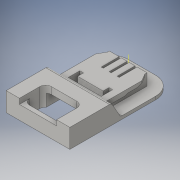
# Autodesk Inventor part: gehaeuse
Saved by Autodesk Inventor 2016 (Build 200138000, 138)
## iProperties
Created: 2016-06-09
Part Number: gehaeuse
Material: Generic
Document SubType Name: Modeling
Designer: Chris
Density: 1 g/cm^3
Appearance: Default
Author: Chris
Autodesk Inventor part; units mm, degrees
ref_plane "YZ Plane" through (0, 0, 0) normal (1, 0, 0) x (0, 1, 0)
ref_plane "XZ Plane" through (0, 0, 0) normal (0, 1, 0) x (-1, 0, 0)
sketch "Sketch1" plane through (0, 0, 0) normal (0, 0, 1) x (1, 0, 0)
  line L0 (-17.75, 0) -> (17.75, 0)
  line L1 (17.75, 0) -> (17.75, -85)
  line L2 (17.75, -85) -> (-17.75, -85)
  line L3 (-17.75, -85) -> (-17.75, 0)
  point P0 (0, 0)
  point P1 (0, 0)
  dimension "d0" = 35.5
  dimension "d1" = 85
  constraints: 8 end point, 2 parallel, 1 coincident, 1 horizontal, 1 midpoint, 1 perpendicular
  measures "d0" distance of L1.end L2.end
  measures "d1" distance of L0.end L1.end
extrude "Extrusion1" add sketch "Sketch1" along normal blind 11
sketch "Sketch2" plane through (0, 0, 0) normal (1, 0, 0) x (0, 1, 0)
  line L0 (-85, 0) -> (0, 0) projected
  line L1 (-85, 0) -> (-85, 11) projected
  line L2 (0, 11) -> (-85, 11) projected
  line L3 (0, 0) -> (0, 11) projected
  line L4 (-85, 82.7102) -> (-37.2472, 0)
  line L5 (0, 0) -> (0, 11) projected
  line L6 (0, 9) -> (-9, 9)
  line L7 (-9, 9) -> (-13.1212, 7.5)
  line L8 (-13.1212, 7.5) -> (-22, 7.5)
  line L9 (-22, 7.5) -> (-24.7475, 6.5)
  line L10 (-24.7475, 6.5) -> (-41, 6.5)
  line L11 (-45.9075, 15) -> (-85, 15)
  line L12 (-85, 15) -> (-85, 11)
  point P0 (-43.5981, 11)
  dimension "d6" = 60
  dimension "d7" = 20
  dimension "d8" = 2
  dimension "d9" = 3.5
  dimension "d10" = 4.5
  dimension "d11" = 6.5
  dimension "d12" = 9
  dimension "d13" = 13.1212
  dimension "d14" = 24.7475
  dimension "d15" = 22
  dimension "d16" = 41
  dimension "d25" = 15
  dimension "d26" = 4
  constraints: 16 end point, 8 point on line, 3 parallel, 3 perpendicular
  measures "d6" angle of L0 L4
  measures "d7" angle of L6 L7
  measures "d8" distance between parallel lines of L2 L6
  measures "d9" distance between parallel lines of L2 L8
  measures "d10" distance between parallel lines of L2 L10
  measures "d11" distance between parallel lines of L0 L10
  measures "d12" distance from line of L3 L6.end
  measures "d13" distance from line of L3 L7.end
  measures "d14" distance from line of L3 L9.end
  measures "d15" distance from line of L3 L8.end
  measures "d16" distance from line of L3 L10.end
  measures "d25" distance between parallel lines of L0 L11
  measures "d26" distance between parallel lines of L11 L2
extrude "Extrusion2" add sketch "Sketch2" along normal mid plane 60 contours L1 L2 L4 L0 | L12 L11 L4 L2
extrude "Extrusion4" add sketch "Sketch2" along normal mid plane 43.6 contours L4 L2 L3 L6 L7 L8 L9 L10
sketch "Sketch3" plane through (0, 0, 0) normal (0, 0, 1) x (1, 0, 0)
  line L0 (-13, 13) -> (13, 13)
  line L1 (-17.75, 0) -> (17.75, 0) projected
  line L2 (-30, -37.2472) -> (-30, -85) projected
  line L3 (30, -85) -> (30, -37.2472) projected
  line L4 (30, -85) -> (-30, -85) projected
  arc A0 (-13, 13) -> (-30, -4) centre (-13, -4) ccw
  arc A1 (30, -4) -> (13, 13) centre (13, -4) ccw
  line L5 (-30, -37.2472) -> (-30, -4)
  line L6 (30, -37.2472) -> (30, -4)
  point P0 (0, 0)
  dimension "d28" = 13
  dimension "d29" = 17
  constraints: 6 end point, 4 point on circle, 4 tangent, 2 centre point, 2 vertical, 1 equal radius, 1 horizontal
  measures "d28" distance between parallel lines of L0 L1
  measures "d29" radius of A0
extrude "Extrusion5" add sketch "Sketch3" against normal blind 3
fillet "Fillet1" radius 3 1 edges at (0, -45.9075, 15)
fillet "Fillet2" radius 2 2 edges at (23.875, -37.2472, 0) (-23.875, -37.2472, 0)
sketch "Sketch4" plane through (0, 0, 11) normal (0, 0, 1) x (1, 0, 0)
  line L0 (21.8, -43.5981) -> (-21.8, -43.5981) projected
  line L1 (21.8, 0) -> (21.8, -43.5981) projected
  line L2 (21.8, 0) -> (-21.8, 0) projected
  line L3 (-21.8, -43.5981) -> (-21.8, 0) projected
  line L4 (-21.8, -43.5981) -> (-21.8, 0) projected
  line L5 (-21.8, -9) -> (-17.75, -2)
  line L6 (-21.8, -9) -> (-13.7128, -9) construction
  line L7 (-17.75, -2) -> (-17.75, 0)
  line L8 (21.8, 0) -> (-21.8, 0) projected
  point P0 (0, 0)
  dimension "d34" = 2
  constraints: 6 end point, 2 point on line, 1 equal length, 1 horizontal, 1 perpendicular
  measures "d34" distance of L7.end L5.end
extrude "Extrusion6" cut sketch "Sketch4" against normal up to next contours L3 L2 L7 L5
mirror "Mirror1" about plane through (0, 0, 0) normal (1, 0, 0) of "Extrusion6"
sketch "Sketch5" plane through (0, 0, 11) normal (0, 0, 1) x (1, 0, 0)
  line L0 (0.95, 0) -> (-0.95, 0)
  line L1 (-0.95, 0) -> (-0.95, -17)
  line L2 (-0.95, -17) -> (0.95, -17)
  line L3 (0.95, -17) -> (0.95, 0)
  line L4 (8.45, 0) -> (6.55, 0)
  line L5 (6.55, 0) -> (6.55, -17)
  line L6 (6.55, -17) -> (8.45, -17)
  line L7 (8.45, -17) -> (8.45, 0)
  line L8 (-6.55, 0) -> (-8.45, 0)
  line L9 (-8.45, 0) -> (-8.45, -17)
  line L10 (-8.45, -17) -> (-6.55, -17)
  line L11 (-6.55, -17) -> (-6.55, 0)
  line L12 (17.75, 0) -> (-17.75, 0) projected
  point P0 (0, 0)
  point P1 (7.5, 0)
  point P2 (-7.5, 0)
  point P3 (0, 0)
  dimension "d37" = 7.5
  dimension "d38" = 7.5
  dimension "d39" = 1.9
  dimension "d40" = 17
  constraints: 24 end point, 6 parallel, 4 midpoint, 3 collinear, 3 horizontal, 3 perpendicular, 3 point on line
  measures "d37" distance of point (0, 0) point (7.5, 0)
  measures "d38" distance of point (0, 0) point (-7.5, 0)
  measures "d39" distance of L1.end L2.end
  measures "d40" distance of L6.end L4.start
extrude "Extrusion7" cut sketch "Sketch5" against normal up to surface (14 mm away)
ref_plane "Work Plane1" through (0, 0, 8) normal (0, 0, 1) x (1, 0, 0)
sketch "Sketch8" plane through (-30, -85, 15) normal (0, 0, 1) x (1, 0, 0)
  line L0 (14.5, 54.9) -> (14.5, 44)
  line L1 (14.5, 44) -> (45.5, 44)
  line L2 (45.5, 44) -> (45.5, 54.9)
  line L3 (45.5, 54.9) -> (42, 54.9)
  line L4 (42, 54.9) -> (42, 49.35)
  line L5 (42, 49.35) -> (18, 49.35)
  line L6 (18, 49.35) -> (18, 54.9)
  line L7 (18, 54.9) -> (14.5, 54.9)
  line L8 (12.5, 4.1) -> (47.5, 4.1)
  line L9 (47.5, 4.1) -> (47.5, 24.6)
  line L10 (47.5, 24.6) -> (12.5, 24.6)
  line L11 (12.5, 24.6) -> (12.5, 4.1)
  arc A0 (12.5, 9.6) -> (18, 4.1) centre (18, 9.6) ccw
  arc A1 (18, 24.6) -> (12.5, 19.1) centre (18, 19.1) ccw
  arc A2 (42, 4.1) -> (47.5, 9.6) centre (42, 9.6) ccw
  arc A3 (47.5, 19.1) -> (42, 24.6) centre (42, 19.1) ccw
  line L12 (12.5, 4.1) -> (12.5, 0)
  line L13 (0, 0) -> (60, 0) projected
  line L14 (47.5, 4.1) -> (47.5, 0)
  point P0 (30, 85)
  point P1 (30, 44)
  point P2 (30, 24.6)
  dimension "d59" = 41
  dimension "d60" = 31
  dimension "d61" = 5.35
  dimension "d62" = 10.9
  dimension "d63" = 3.5
  dimension "d64" = 19.4
  dimension "d65" = 35
  dimension "d66" = 20.5
  dimension "d67" = 5.5
  constraints: 28 end point, 11 point on line, 8 point on circle, 8 tangent, 7 perpendicular, 4 centre point, 4 parallel, 3 equal radius, 2 midpoint, 2 vertical, 2 vertical alignment, 1 collinear, 1 horizontal
  measures "d59" distance from line of point (30, 85) L1
  measures "d60" distance of L0.end L1.end
  measures "d61" distance between parallel lines of L1 L5
  measures "d62" distance between parallel lines of L1 L7
  measures "d63" distance of L6.end L0.start
  measures "d64" distance between parallel lines of L10 L1
  measures "d65" distance of L9.end L10.end
  measures "d66" distance of L10.end L8.start
  measures "d67" radius of A0
extrude "Extrusion11" cut sketch "Sketch8" along normal through all both and the other way through all contours L7 L6 L5 L4 L3 L2 L1 L0 | A0 L11 A1 L10 A3 L9 A2 L8
extrude "Extrusion12" cut sketch "Sketch8" against normal blind 5 contours L11 A0 L8 | L8 L14 L13 L12 | A2 L9 L8
sketch "Sketch9" plane through (0, 0, -3) normal (0, 0, -1) x (-1, 0, 0)
  line L0 (15.5, -41) -> (-15.5, -41) projected
  line L1 (-12, -60.4) -> (12, -60.4) projected
  arc A0 (17.5, -65.9) -> (12, -60.4) centre (12, -65.9) ccw projected
  arc A1 (-12, -60.4) -> (-17.5, -65.9) centre (-12, -65.9) ccw projected
  line L2 (15.5, -41) -> (15.5, -61.6574)
  line L3 (30, -37.8246) -> (17.75, -37.8246) projected
  line L4 (-15.5, -41) -> (-15.5, -61.6574)
  point P0 (0, 0)
  constraints: 4 end point, 2 point on circle, 1 parallel, 1 perpendicular
extrude "Extrusion13" cut sketch "Sketch9" against normal blind 11.5
equation "\"overprint\" = 0.1"
body "Solid1"
